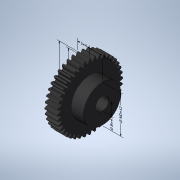
# Autodesk Inventor part: 21104000
Saved by Autodesk Inventor 2021 (Build 250183000, 183)
## iProperties
Created: 2025-12-15
Part Number: 21104000
Material: Generic
Catalog Web Link: www.3dfindit.com
Description: MAE-STZR-M0.5-MN-B4-ST-Spur Gears Made from Steel, with One-Sided Hub, Module 0.5, Tooth Width 4 mm
Vendor: MAEDLER
Document SubType Name: Modeling
Designer: psAdmin
Manufacturer: MAEDLER
Mass: 12 g
Surface Area: 13.391 cm^2
Volume: 1.60041 cm^3
Density: 1 g/cm^3
Appearance: PSOLRGB-176-176-176
Category: PARTsolutions
Company: MAEDLER
Title: 21104000
Author: Cadenas PARTsolutions
Comments: Spur Gears Made from Steel, with One-Sided Hub, Module 0.5, Tooth Width 4 mm
PSOL_IDENT_0: {$CADENAS_DATA/23d-libs/maedler/antriebselemente/stirnzahnraeder/stirnzahnraeder_stahl/modul_0_5_und
PSOL_IDENT_1: _0_7/stzr_m_0_5_zb4_st_mn.prj},173 {VTYP=3D},{NB=21104000},{LINA=21104000},{NN=MAE-STZR-M0.5-MN-B4-S
PSOL_IDENT_2: T},{DATE=31.10.2024 07:34:43},{GEOMDATE=31.10.2024 07:34:43},{VERSION=},{LINEID=240},{WBVAR=},{WBNUM
PSOL_IDENT_3: ERIC=}  {NB=21104000},{LINA=21104000},{KT=DUMMY},{ARTNR=21104000},{WEBSHOP=Produktdetails / Katalogs
PSOL_IDENT_4: eite / Montageanleitung},{MATK=Stahl},{MAT=Stahl 11SMn30+C (1.0715)},{M=0.5},{Z=40},{B=4},{DA=21.0},
PSOL_IDENT_5: {D=20.0},{NL=4},{ND=12},{BH7=4},{MD=10.3},{GEW=12.0},{CTN=84839089},{DIST=0.967},{GKD=18.79385},{FKD=
PSOL_IDENT_6: 18.83300},{T0=1.57080},{UF=62.83185},{TLG=1.57080},{A=3.42020},{A3=1.14007},{PI=0.39270},{R2=0.04},{
PSOL_IDENT_7: CNSDWTEMPLATE=_dw/ansicht_right_front.dw}
NB: 21104000
NN: MAE-STZR-M0.5-MN-B4-ST
NT: Spur Gears Made from Steel, with One-Sided Hub, Module 0.5, Tooth Width 4 mm
NBSYN: $ARTNR.
LINA: 21104000
CATALOG: MÄDLER
ARTNR: 21104000
WEBSHOP: Product details / Catalogue page / Assembly instructions
MATK: Steel
MAT: Steel 11SMn30+C (1.0715)
M: 0.5
Z: 40
B: 4
DA: 21
D: 20
NL: 4
ND: 12
BH7: 4
MD: 10.3
GEW: 12
CTN: 84839089
SUPPLIER: MAEDLER
ARTICLENO: 21104000
BOMINFO: 21104000
CREATOR: CADENAS GmbH
Autodesk Inventor part; units mm, degrees
ref_plane "YZ Plane" through (0, 0, 0) normal (1, 0, 0) x (0, 1, 0)
ref_plane "XZ Plane" through (0, 0, 0) normal (0, 1, 0) x (-1, 0, 0)
ref_plane "XY Plane" through (0, 0, 0) normal (0, 0, 1) x (1, 0, 0)
sketch "Sketch_2" plane through (0, 0, 0) normal (0, 0, 1) x (1, 0, 0)
  line L0 (6, 0) -> (-2, 0)
  line L1 (-2, 10.5) -> (-2, 2.1414)
  line L2 (-2, 2.1414) -> (-1.8586, 2)
  line L3 (-1.8586, 2) -> (5.8586, 2)
  line L4 (5.8586, 2) -> (6, 2.1414)
  line L5 (6, 2.1414) -> (6, 5.8586)
  line L6 (6, 5.8586) -> (5.8586, 6)
  line L7 (5.8586, 6) -> (2.1, 6)
  arc A0 (2, 6.1) -> (2.1, 6) centre (2.1, 6.1) ccw
  line L8 (2, 6.1) -> (2, 10.5)
  line L9 (2, 10.5) -> (-2, 10.5)
  constraints: 20 end point, 2 point on circle, 1 centre point
revolve "Revolution1" add sketch "Sketch_2" angle 360 about axis through (6, 0, 0) along (1, 0, 0)
sketch "Sketch_4" plane through (0, 0, 0) normal (1, 0, 0) x (0, 0, -1)
  circle A0 centre (0, 0) radius 21
  arc A1 (-10.4983, 0.1884) -> (-10.4983, -0.1884) centre (0, 0) ccw
  arc A2 (-10.4983, -0.1884) -> (-10.1352, -0.3434) centre (-8.8221, 3.2362) ccw
  arc A3 (-10.1352, -0.3434) -> (-9.9923, -0.3926) centre (-8.9496, 2.8648) ccw
  arc A4 (-9.9923, -0.3926) -> (-9.4352, -0.5161) centre (-9.0615, 2.4884) ccw
  arc A5 (-9.4002, -0.5534) -> (-9.4352, -0.5161) centre (-9.4402, -0.5558) ccw
  arc A6 (-9.4002, -0.5534) -> (-9.3711, -0.9239) centre (0, 0) ccw
  arc A7 (-9.3998, -0.9663) -> (-9.3711, -0.9239) centre (-9.4109, -0.9278) ccw
  arc A8 (-9.3998, -0.9663) -> (-9.9307, -1.1754) centre (-8.5606, -3.8753) ccw
  arc A9 (-9.9307, -1.1754) -> (-10.0641, -1.2464) centre (-8.3913, -4.2295) ccw
  arc A10 (-10.0641, -1.2464) -> (-10.3985, -1.4562) centre (-8.2072, -4.5764) ccw
  arc A11 (-10.3985, -1.4562) -> (-10.3396, -1.8283) centre (0, 0) ccw
  arc A12 (-10.3396, -1.8283) -> (-9.9567, -1.9246) centre (-9.2197, 1.8163) ccw
  arc A13 (-9.9567, -1.9246) -> (-9.8079, -1.9509) centre (-9.2876, 1.4295) ccw
  arc A14 (-9.8079, -1.9509) -> (-9.2383, -1.9857) centre (-9.3392, 1.0402) ccw
  arc A15 (-9.1979, -2.0171) -> (-9.2383, -1.9857) centre (-9.237, -2.0257) ccw
  arc A16 (-9.1979, -2.0171) -> (-9.1112, -2.3785) centre (0, 0) ccw
  arc A17 (-9.1329, -2.4248) -> (-9.1112, -2.3785) centre (-9.1499, -2.3886) ccw
  arc A18 (-9.1329, -2.4248) -> (-9.6246, -2.7144) centre (-7.849, -5.1667) ccw
  arc A19 (-9.6246, -2.7144) -> (-9.7452, -2.8054) centre (-7.6263, -5.4902) ccw
  arc A20 (-9.7452, -2.8054) -> (-10.0427, -3.065) centre (-7.3903, -5.804) ccw
  arc A21 (-10.0427, -3.065) -> (-9.9263, -3.4233) centre (0, 0) ccw
  arc A22 (-9.9263, -3.4233) -> (-9.533, -3.4585) centre (-9.3903, 0.3516) ccw
  arc A23 (-9.533, -3.4585) -> (-9.3819, -3.4612) centre (-9.3968, -0.041) ccw
  arc A24 (-9.3819, -3.4612) -> (-8.8139, -3.4065) centre (-9.3869, -0.4336) ccw
  arc A25 (-8.7691, -3.4312) -> (-8.8139, -3.4065) centre (-8.8064, -3.4457) ccw
  arc A26 (-8.7691, -3.4312) -> (-8.6269, -3.7745) centre (0, 0) ccw
  arc A27 (-8.6411, -3.8237) -> (-8.6269, -3.7745) centre (-8.6636, -3.7905) ccw
  arc A28 (-8.6411, -3.8237) -> (-9.0814, -4.1866) centre (-6.9441, -6.331) ccw
  arc A29 (-9.0814, -4.1866) -> (-9.1864, -4.2953) centre (-6.6736, -6.6156) ccw
  arc A30 (-9.1864, -4.2953) -> (-9.4396, -4.5983) centre (-6.3913, -6.8886) ccw
  arc A31 (-9.4396, -4.5983) -> (-9.2685, -4.934) centre (0, 0) ccw
  arc A32 (-9.2685, -4.934) -> (-8.8746, -4.9072) centre (-9.3297, -1.1217) ccw
  arc A33 (-8.8746, -4.9072) -> (-8.725, -4.8862) centre (-9.2747, -1.5105) ccw
  arc A34 (-8.725, -4.8862) -> (-8.1725, -4.7433) centre (-9.2035, -1.8967) ccw
  arc A35 (-8.1244, -4.7607) -> (-8.1725, -4.7433) centre (-8.1589, -4.7809) ccw
  arc A36 (-8.1244, -4.7607) -> (-7.9302, -5.0776) centre (0, 0) ccw
  arc A37 (-7.9366, -5.1284) -> (-7.9302, -5.0776) centre (-7.9639, -5.0992) ccw
  arc A38 (-7.9366, -5.1284) -> (-8.3147, -5.5557) centre (-5.8683, -7.3393) ccw
  arc A39 (-8.3147, -5.5557) -> (-8.4013, -5.6795) centre (-5.5565, -7.5781) ccw
  arc A40 (-8.4013, -5.6795) -> (-8.604, -6.0184) centre (-5.235, -7.8036) ccw
  arc A41 (-8.604, -6.0184) -> (-8.3826, -6.3231) centre (0, 0) ccw
  arc A42 (-8.3826, -6.3231) -> (-7.9977, -6.2351) centre (-9.0394, -2.5673) ccw
  arc A43 (-7.9977, -6.2351) -> (-7.8532, -6.1909) centre (-8.9243, -2.9428) ccw
  arc A44 (-7.8532, -6.1909) -> (-7.3299, -5.9634) centre (-8.7935, -3.3131) ccw
  arc A45 (-7.2796, -5.973) -> (-7.3299, -5.9634) centre (-7.3106, -5.9984) ccw
  arc A46 (-7.2796, -5.973) -> (-7.0383, -6.2556) centre (0, 0) ccw
  arc A47 (-7.0366, -6.3068) -> (-7.0383, -6.2556) centre (-7.0682, -6.2822) ccw
  arc A48 (-7.0366, -6.3068) -> (-7.3432, -6.788) centre (-4.6479, -8.167) ccw
  arc A49 (-7.3432, -6.788) -> (-7.4094, -6.9239) centre (-4.3026, -8.354) ccw
  arc A50 (-7.4094, -6.9239) -> (-7.5566, -7.2902) centre (-3.9498, -8.5265) ccw
  arc A51 (-7.5566, -7.2902) -> (-7.2902, -7.5566) centre (0, 0) ccw
  arc A52 (-7.2902, -7.5566) -> (-6.9239, -7.4094) centre (-8.5265, -3.9498) ccw
  arc A53 (-6.9239, -7.4094) -> (-6.788, -7.3432) centre (-8.354, -4.3026) ccw
  arc A54 (-6.788, -7.3432) -> (-6.3068, -7.0366) centre (-8.167, -4.6479) ccw
  arc A55 (-6.2556, -7.0383) -> (-6.3068, -7.0366) centre (-6.2822, -7.0682) ccw
  arc A56 (-6.2556, -7.0383) -> (-5.973, -7.2796) centre (0, 0) ccw
  arc A57 (-5.9634, -7.3299) -> (-5.973, -7.2796) centre (-5.9984, -7.3106) ccw
  arc A58 (-5.9634, -7.3299) -> (-6.1909, -7.8532) centre (-3.3131, -8.7935) ccw
  arc A59 (-6.1909, -7.8532) -> (-6.2351, -7.9977) centre (-2.9428, -8.9243) ccw
  arc A60 (-6.2351, -7.9977) -> (-6.3231, -8.3826) centre (-2.5673, -9.0394) ccw
  arc A61 (-6.3231, -8.3826) -> (-6.0184, -8.604) centre (0, 0) ccw
  arc A62 (-6.0184, -8.604) -> (-5.6795, -8.4013) centre (-7.8036, -5.235) ccw
  arc A63 (-5.6795, -8.4013) -> (-5.5557, -8.3147) centre (-7.5781, -5.5565) ccw
  arc A64 (-5.5557, -8.3147) -> (-5.1284, -7.9366) centre (-7.3393, -5.8683) ccw
  arc A65 (-5.0776, -7.9302) -> (-5.1284, -7.9366) centre (-5.0992, -7.9639) ccw
  arc A66 (-5.0776, -7.9302) -> (-4.7607, -8.1244) centre (0, 0) ccw
  arc A67 (-4.7433, -8.1725) -> (-4.7607, -8.1244) centre (-4.7809, -8.1589) ccw
  arc A68 (-4.7433, -8.1725) -> (-4.8862, -8.725) centre (-1.8967, -9.2035) ccw
  arc A69 (-4.8862, -8.725) -> (-4.9072, -8.8746) centre (-1.5105, -9.2747) ccw
  arc A70 (-4.9072, -8.8746) -> (-4.934, -9.2685) centre (-1.1217, -9.3297) ccw
  arc A71 (-4.934, -9.2685) -> (-4.5983, -9.4396) centre (0, 0) ccw
  arc A72 (-4.5983, -9.4396) -> (-4.2953, -9.1864) centre (-6.8886, -6.3913) ccw
  arc A73 (-4.2953, -9.1864) -> (-4.1866, -9.0814) centre (-6.6156, -6.6736) ccw
  arc A74 (-4.1866, -9.0814) -> (-3.8237, -8.6411) centre (-6.331, -6.9441) ccw
  arc A75 (-3.7745, -8.6269) -> (-3.8237, -8.6411) centre (-3.7905, -8.6636) ccw
  arc A76 (-3.7745, -8.6269) -> (-3.4312, -8.7691) centre (0, 0) ccw
  arc A77 (-3.4065, -8.8139) -> (-3.4312, -8.7691) centre (-3.4457, -8.8064) ccw
  arc A78 (-3.4065, -8.8139) -> (-3.4612, -9.3819) centre (-0.4336, -9.3869) ccw
  arc A79 (-3.4612, -9.3819) -> (-3.4585, -9.533) centre (-0.041, -9.3968) ccw
  arc A80 (-3.4585, -9.533) -> (-3.4233, -9.9263) centre (0.3516, -9.3903) ccw
  arc A81 (-3.4233, -9.9263) -> (-3.065, -10.0427) centre (0, 0) ccw
  arc A82 (-3.065, -10.0427) -> (-2.8054, -9.7452) centre (-5.804, -7.3903) ccw
  arc A83 (-2.8054, -9.7452) -> (-2.7144, -9.6246) centre (-5.4902, -7.6263) ccw
  arc A84 (-2.7144, -9.6246) -> (-2.4248, -9.1329) centre (-5.1667, -7.849) ccw
  arc A85 (-2.3785, -9.1112) -> (-2.4248, -9.1329) centre (-2.3886, -9.1499) ccw
  arc A86 (-2.3785, -9.1112) -> (-2.0171, -9.1979) centre (0, 0) ccw
  arc A87 (-1.9857, -9.2383) -> (-2.0171, -9.1979) centre (-2.0257, -9.237) ccw
  arc A88 (-1.9857, -9.2383) -> (-1.9509, -9.8079) centre (1.0402, -9.3392) ccw
  arc A89 (-1.9509, -9.8079) -> (-1.9246, -9.9567) centre (1.4295, -9.2876) ccw
  arc A90 (-1.9246, -9.9567) -> (-1.8283, -10.3396) centre (1.8163, -9.2197) ccw
  arc A91 (-1.8283, -10.3396) -> (-1.4562, -10.3985) centre (0, 0) ccw
  arc A92 (-1.4562, -10.3985) -> (-1.2464, -10.0641) centre (-4.5764, -8.2072) ccw
  arc A93 (-1.2464, -10.0641) -> (-1.1754, -9.9307) centre (-4.2295, -8.3913) ccw
  arc A94 (-1.1754, -9.9307) -> (-0.9663, -9.3998) centre (-3.8753, -8.5606) ccw
  arc A95 (-0.9239, -9.3711) -> (-0.9663, -9.3998) centre (-0.9278, -9.4109) ccw
  arc A96 (-0.9239, -9.3711) -> (-0.5534, -9.4002) centre (0, 0) ccw
  arc A97 (-0.5161, -9.4352) -> (-0.5534, -9.4002) centre (-0.5558, -9.4402) ccw
  arc A98 (-0.5161, -9.4352) -> (-0.3926, -9.9923) centre (2.4884, -9.0615) ccw
  arc A99 (-0.3926, -9.9923) -> (-0.3434, -10.1352) centre (2.8648, -8.9496) ccw
  arc A100 (-0.3434, -10.1352) -> (-0.1884, -10.4983) centre (3.2362, -8.8221) ccw
  arc A101 (-0.1884, -10.4983) -> (0.1884, -10.4983) centre (0, 0) ccw
  arc A102 (0.1884, -10.4983) -> (0.3434, -10.1352) centre (-3.2362, -8.8221) ccw
  arc A103 (0.3434, -10.1352) -> (0.3926, -9.9923) centre (-2.8648, -8.9496) ccw
  arc A104 (0.3926, -9.9923) -> (0.5161, -9.4352) centre (-2.4884, -9.0615) ccw
  arc A105 (0.5534, -9.4002) -> (0.5161, -9.4352) centre (0.5558, -9.4402) ccw
  arc A106 (0.5534, -9.4002) -> (0.9239, -9.3711) centre (0, 0) ccw
  arc A107 (0.9663, -9.3998) -> (0.9239, -9.3711) centre (0.9278, -9.4109) ccw
  arc A108 (0.9663, -9.3998) -> (1.1754, -9.9307) centre (3.8753, -8.5606) ccw
  arc A109 (1.1754, -9.9307) -> (1.2464, -10.0641) centre (4.2295, -8.3913) ccw
  arc A110 (1.2464, -10.0641) -> (1.4562, -10.3985) centre (4.5764, -8.2072) ccw
  arc A111 (1.4562, -10.3985) -> (1.8283, -10.3396) centre (0, 0) ccw
  arc A112 (1.8283, -10.3396) -> (1.9246, -9.9567) centre (-1.8163, -9.2197) ccw
  arc A113 (1.9246, -9.9567) -> (1.9509, -9.8079) centre (-1.4295, -9.2876) ccw
  arc A114 (1.9509, -9.8079) -> (1.9857, -9.2383) centre (-1.0402, -9.3392) ccw
  arc A115 (2.0171, -9.1979) -> (1.9857, -9.2383) centre (2.0257, -9.237) ccw
  arc A116 (2.0171, -9.1979) -> (2.3785, -9.1112) centre (0, 0) ccw
  arc A117 (2.4248, -9.1329) -> (2.3785, -9.1112) centre (2.3886, -9.1499) ccw
  arc A118 (2.4248, -9.1329) -> (2.7144, -9.6246) centre (5.1667, -7.849) ccw
  arc A119 (2.7144, -9.6246) -> (2.8054, -9.7452) centre (5.4902, -7.6263) ccw
  arc A120 (2.8054, -9.7452) -> (3.065, -10.0427) centre (5.804, -7.3903) ccw
  arc A121 (3.065, -10.0427) -> (3.4233, -9.9263) centre (0, 0) ccw
  arc A122 (3.4233, -9.9263) -> (3.4585, -9.533) centre (-0.3516, -9.3903) ccw
  arc A123 (3.4585, -9.533) -> (3.4612, -9.3819) centre (0.041, -9.3968) ccw
  arc A124 (3.4612, -9.3819) -> (3.4065, -8.8139) centre (0.4336, -9.3869) ccw
  arc A125 (3.4312, -8.7691) -> (3.4065, -8.8139) centre (3.4457, -8.8064) ccw
  arc A126 (3.4312, -8.7691) -> (3.7745, -8.6269) centre (0, 0) ccw
  arc A127 (3.8237, -8.6411) -> (3.7745, -8.6269) centre (3.7905, -8.6636) ccw
  arc A128 (3.8237, -8.6411) -> (4.1866, -9.0814) centre (6.331, -6.9441) ccw
  arc A129 (4.1866, -9.0814) -> (4.2953, -9.1864) centre (6.6156, -6.6736) ccw
  arc A130 (4.2953, -9.1864) -> (4.5983, -9.4396) centre (6.8886, -6.3913) ccw
  arc A131 (4.5983, -9.4396) -> (4.934, -9.2685) centre (0, 0) ccw
  arc A132 (4.934, -9.2685) -> (4.9072, -8.8746) centre (1.1217, -9.3297) ccw
  arc A133 (4.9072, -8.8746) -> (4.8862, -8.725) centre (1.5105, -9.2747) ccw
  arc A134 (4.8862, -8.725) -> (4.7433, -8.1725) centre (1.8967, -9.2035) ccw
  arc A135 (4.7607, -8.1244) -> (4.7433, -8.1725) centre (4.7809, -8.1589) ccw
  arc A136 (4.7607, -8.1244) -> (5.0776, -7.9302) centre (0, 0) ccw
  arc A137 (5.1284, -7.9366) -> (5.0776, -7.9302) centre (5.0992, -7.9639) ccw
  arc A138 (5.1284, -7.9366) -> (5.5557, -8.3147) centre (7.3393, -5.8683) ccw
  arc A139 (5.5557, -8.3147) -> (5.6795, -8.4013) centre (7.5781, -5.5565) ccw
  arc A140 (5.6795, -8.4013) -> (6.0184, -8.604) centre (7.8036, -5.235) ccw
  arc A141 (6.0184, -8.604) -> (6.3231, -8.3826) centre (0, 0) ccw
  arc A142 (6.3231, -8.3826) -> (6.2351, -7.9977) centre (2.5673, -9.0394) ccw
  arc A143 (6.2351, -7.9977) -> (6.1909, -7.8532) centre (2.9428, -8.9243) ccw
  arc A144 (6.1909, -7.8532) -> (5.9634, -7.3299) centre (3.3131, -8.7935) ccw
  arc A145 (5.973, -7.2796) -> (5.9634, -7.3299) centre (5.9984, -7.3106) ccw
  arc A146 (5.973, -7.2796) -> (6.2556, -7.0383) centre (0, 0) ccw
  arc A147 (6.3068, -7.0366) -> (6.2556, -7.0383) centre (6.2822, -7.0682) ccw
  arc A148 (6.3068, -7.0366) -> (6.788, -7.3432) centre (8.167, -4.6479) ccw
  arc A149 (6.788, -7.3432) -> (6.9239, -7.4094) centre (8.354, -4.3026) ccw
  arc A150 (6.9239, -7.4094) -> (7.2902, -7.5566) centre (8.5265, -3.9498) ccw
  arc A151 (7.2902, -7.5566) -> (7.5566, -7.2902) centre (0, 0) ccw
  arc A152 (7.5566, -7.2902) -> (7.4094, -6.9239) centre (3.9498, -8.5265) ccw
  arc A153 (7.4094, -6.9239) -> (7.3432, -6.788) centre (4.3026, -8.354) ccw
  arc A154 (7.3432, -6.788) -> (7.0366, -6.3068) centre (4.6479, -8.167) ccw
  arc A155 (7.0383, -6.2556) -> (7.0366, -6.3068) centre (7.0682, -6.2822) ccw
  arc A156 (7.0383, -6.2556) -> (7.2796, -5.973) centre (0, 0) ccw
  arc A157 (7.3299, -5.9634) -> (7.2796, -5.973) centre (7.3106, -5.9984) ccw
  arc A158 (7.3299, -5.9634) -> (7.8532, -6.1909) centre (8.7935, -3.3131) ccw
  arc A159 (7.8532, -6.1909) -> (7.9977, -6.2351) centre (8.9243, -2.9428) ccw
  arc A160 (7.9977, -6.2351) -> (8.3826, -6.3231) centre (9.0394, -2.5673) ccw
  arc A161 (8.3826, -6.3231) -> (8.604, -6.0184) centre (0, 0) ccw
  arc A162 (8.604, -6.0184) -> (8.4013, -5.6795) centre (5.235, -7.8036) ccw
  arc A163 (8.4013, -5.6795) -> (8.3147, -5.5557) centre (5.5565, -7.5781) ccw
  arc A164 (8.3147, -5.5557) -> (7.9366, -5.1284) centre (5.8683, -7.3393) ccw
  arc A165 (7.9302, -5.0776) -> (7.9366, -5.1284) centre (7.9639, -5.0992) ccw
  arc A166 (7.9302, -5.0776) -> (8.1244, -4.7607) centre (0, 0) ccw
  arc A167 (8.1725, -4.7433) -> (8.1244, -4.7607) centre (8.1589, -4.7809) ccw
  arc A168 (8.1725, -4.7433) -> (8.725, -4.8862) centre (9.2035, -1.8967) ccw
  arc A169 (8.725, -4.8862) -> (8.8746, -4.9072) centre (9.2747, -1.5105) ccw
  arc A170 (8.8746, -4.9072) -> (9.2685, -4.934) centre (9.3297, -1.1217) ccw
  arc A171 (9.2685, -4.934) -> (9.4396, -4.5983) centre (0, 0) ccw
  arc A172 (9.4396, -4.5983) -> (9.1864, -4.2953) centre (6.3913, -6.8886) ccw
  arc A173 (9.1864, -4.2953) -> (9.0814, -4.1866) centre (6.6736, -6.6156) ccw
  arc A174 (9.0814, -4.1866) -> (8.6411, -3.8237) centre (6.9441, -6.331) ccw
  arc A175 (8.6269, -3.7745) -> (8.6411, -3.8237) centre (8.6636, -3.7905) ccw
  arc A176 (8.6269, -3.7745) -> (8.7691, -3.4312) centre (0, 0) ccw
  arc A177 (8.8139, -3.4065) -> (8.7691, -3.4312) centre (8.8064, -3.4457) ccw
  arc A178 (8.8139, -3.4065) -> (9.3819, -3.4612) centre (9.3869, -0.4336) ccw
  arc A179 (9.3819, -3.4612) -> (9.533, -3.4585) centre (9.3968, -0.041) ccw
  arc A180 (9.533, -3.4585) -> (9.9263, -3.4233) centre (9.3903, 0.3516) ccw
  arc A181 (9.9263, -3.4233) -> (10.0427, -3.065) centre (0, 0) ccw
  arc A182 (10.0427, -3.065) -> (9.7452, -2.8054) centre (7.3903, -5.804) ccw
  arc A183 (9.7452, -2.8054) -> (9.6246, -2.7144) centre (7.6263, -5.4902) ccw
  arc A184 (9.6246, -2.7144) -> (9.1329, -2.4248) centre (7.849, -5.1667) ccw
  arc A185 (9.1112, -2.3785) -> (9.1329, -2.4248) centre (9.1499, -2.3886) ccw
  arc A186 (9.1112, -2.3785) -> (9.1979, -2.0171) centre (0, 0) ccw
  arc A187 (9.2383, -1.9857) -> (9.1979, -2.0171) centre (9.237, -2.0257) ccw
  arc A188 (9.2383, -1.9857) -> (9.8079, -1.9509) centre (9.3392, 1.0402) ccw
  arc A189 (9.8079, -1.9509) -> (9.9567, -1.9246) centre (9.2876, 1.4295) ccw
  arc A190 (9.9567, -1.9246) -> (10.3396, -1.8283) centre (9.2197, 1.8163) ccw
  arc A191 (10.3396, -1.8283) -> (10.3985, -1.4562) centre (0, 0) ccw
  arc A192 (10.3985, -1.4562) -> (10.0641, -1.2464) centre (8.2072, -4.5764) ccw
  arc A193 (10.0641, -1.2464) -> (9.9307, -1.1754) centre (8.3913, -4.2295) ccw
  arc A194 (9.9307, -1.1754) -> (9.3998, -0.9663) centre (8.5606, -3.8753) ccw
  arc A195 (9.3711, -0.9239) -> (9.3998, -0.9663) centre (9.4109, -0.9278) ccw
  arc A196 (9.3711, -0.9239) -> (9.4002, -0.5534) centre (0, 0) ccw
  arc A197 (9.4352, -0.5161) -> (9.4002, -0.5534) centre (9.4402, -0.5558) ccw
  arc A198 (9.4352, -0.5161) -> (9.9923, -0.3926) centre (9.0615, 2.4884) ccw
  arc A199 (9.9923, -0.3926) -> (10.1352, -0.3434) centre (8.9496, 2.8648) ccw
  arc A200 (10.1352, -0.3434) -> (10.4983, -0.1884) centre (8.8221, 3.2362) ccw
  arc A201 (10.4983, -0.1884) -> (10.4983, 0.1884) centre (0, 0) ccw
  arc A202 (10.4983, 0.1884) -> (10.1352, 0.3434) centre (8.8221, -3.2362) ccw
  arc A203 (10.1352, 0.3434) -> (9.9923, 0.3926) centre (8.9496, -2.8648) ccw
  arc A204 (9.9923, 0.3926) -> (9.4352, 0.5161) centre (9.0615, -2.4884) ccw
  arc A205 (9.4002, 0.5534) -> (9.4352, 0.5161) centre (9.4402, 0.5558) ccw
  arc A206 (9.4002, 0.5534) -> (9.3711, 0.9239) centre (0, 0) ccw
  arc A207 (9.3998, 0.9663) -> (9.3711, 0.9239) centre (9.4109, 0.9278) ccw
  arc A208 (9.3998, 0.9663) -> (9.9307, 1.1754) centre (8.5606, 3.8753) ccw
  arc A209 (9.9307, 1.1754) -> (10.0641, 1.2464) centre (8.3913, 4.2295) ccw
  arc A210 (10.0641, 1.2464) -> (10.3985, 1.4562) centre (8.2072, 4.5764) ccw
  arc A211 (10.3985, 1.4562) -> (10.3396, 1.8283) centre (0, 0) ccw
  arc A212 (10.3396, 1.8283) -> (9.9567, 1.9246) centre (9.2197, -1.8163) ccw
  arc A213 (9.9567, 1.9246) -> (9.8079, 1.9509) centre (9.2876, -1.4295) ccw
  arc A214 (9.8079, 1.9509) -> (9.2383, 1.9857) centre (9.3392, -1.0402) ccw
  arc A215 (9.1979, 2.0171) -> (9.2383, 1.9857) centre (9.237, 2.0257) ccw
  arc A216 (9.1979, 2.0171) -> (9.1112, 2.3785) centre (0, 0) ccw
  arc A217 (9.1329, 2.4248) -> (9.1112, 2.3785) centre (9.1499, 2.3886) ccw
  arc A218 (9.1329, 2.4248) -> (9.6246, 2.7144) centre (7.849, 5.1667) ccw
  arc A219 (9.6246, 2.7144) -> (9.7452, 2.8054) centre (7.6263, 5.4902) ccw
  arc A220 (9.7452, 2.8054) -> (10.0427, 3.065) centre (7.3903, 5.804) ccw
  arc A221 (10.0427, 3.065) -> (9.9263, 3.4233) centre (0, 0) ccw
  arc A222 (9.9263, 3.4233) -> (9.533, 3.4585) centre (9.3903, -0.3516) ccw
  arc A223 (9.533, 3.4585) -> (9.3819, 3.4612) centre (9.3968, 0.041) ccw
  arc A224 (9.3819, 3.4612) -> (8.8139, 3.4065) centre (9.3869, 0.4336) ccw
  arc A225 (8.7691, 3.4312) -> (8.8139, 3.4065) centre (8.8064, 3.4457) ccw
  arc A226 (8.7691, 3.4312) -> (8.6269, 3.7745) centre (0, 0) ccw
  arc A227 (8.6411, 3.8237) -> (8.6269, 3.7745) centre (8.6636, 3.7905) ccw
  arc A228 (8.6411, 3.8237) -> (9.0814, 4.1866) centre (6.9441, 6.331) ccw
  arc A229 (9.0814, 4.1866) -> (9.1864, 4.2953) centre (6.6736, 6.6156) ccw
  arc A230 (9.1864, 4.2953) -> (9.4396, 4.5983) centre (6.3913, 6.8886) ccw
  arc A231 (9.4396, 4.5983) -> (9.2685, 4.934) centre (0, 0) ccw
  arc A232 (9.2685, 4.934) -> (8.8746, 4.9072) centre (9.3297, 1.1217) ccw
  arc A233 (8.8746, 4.9072) -> (8.725, 4.8862) centre (9.2747, 1.5105) ccw
  arc A234 (8.725, 4.8862) -> (8.1725, 4.7433) centre (9.2035, 1.8967) ccw
  arc A235 (8.1244, 4.7607) -> (8.1725, 4.7433) centre (8.1589, 4.7809) ccw
  arc A236 (8.1244, 4.7607) -> (7.9302, 5.0776) centre (0, 0) ccw
  arc A237 (7.9366, 5.1284) -> (7.9302, 5.0776) centre (7.9639, 5.0992) ccw
  arc A238 (7.9366, 5.1284) -> (8.3147, 5.5557) centre (5.8683, 7.3393) ccw
  arc A239 (8.3147, 5.5557) -> (8.4013, 5.6795) centre (5.5565, 7.5781) ccw
  arc A240 (8.4013, 5.6795) -> (8.604, 6.0184) centre (5.235, 7.8036) ccw
  arc A241 (8.604, 6.0184) -> (8.3826, 6.3231) centre (0, 0) ccw
  arc A242 (8.3826, 6.3231) -> (7.9977, 6.2351) centre (9.0394, 2.5673) ccw
  arc A243 (7.9977, 6.2351) -> (7.8532, 6.1909) centre (8.9243, 2.9428) ccw
  arc A244 (7.8532, 6.1909) -> (7.3299, 5.9634) centre (8.7935, 3.3131) ccw
  arc A245 (7.2796, 5.973) -> (7.3299, 5.9634) centre (7.3106, 5.9984) ccw
  arc A246 (7.2796, 5.973) -> (7.0383, 6.2556) centre (0, 0) ccw
  arc A247 (7.0366, 6.3068) -> (7.0383, 6.2556) centre (7.0682, 6.2822) ccw
  arc A248 (7.0366, 6.3068) -> (7.3432, 6.788) centre (4.6479, 8.167) ccw
  arc A249 (7.3432, 6.788) -> (7.4094, 6.9239) centre (4.3026, 8.354) ccw
  arc A250 (7.4094, 6.9239) -> (7.5566, 7.2902) centre (3.9498, 8.5265) ccw
  arc A251 (7.5566, 7.2902) -> (7.2902, 7.5566) centre (0, 0) ccw
  arc A252 (7.2902, 7.5566) -> (6.9239, 7.4094) centre (8.5265, 3.9498) ccw
  arc A253 (6.9239, 7.4094) -> (6.788, 7.3432) centre (8.354, 4.3026) ccw
  arc A254 (6.788, 7.3432) -> (6.3068, 7.0366) centre (8.167, 4.6479) ccw
  arc A255 (6.2556, 7.0383) -> (6.3068, 7.0366) centre (6.2822, 7.0682) ccw
  arc A256 (6.2556, 7.0383) -> (5.973, 7.2796) centre (0, 0) ccw
  arc A257 (5.9634, 7.3299) -> (5.973, 7.2796) centre (5.9984, 7.3106) ccw
  arc A258 (5.9634, 7.3299) -> (6.1909, 7.8532) centre (3.3131, 8.7935) ccw
  arc A259 (6.1909, 7.8532) -> (6.2351, 7.9977) centre (2.9428, 8.9243) ccw
  arc A260 (6.2351, 7.9977) -> (6.3231, 8.3826) centre (2.5673, 9.0394) ccw
  arc A261 (6.3231, 8.3826) -> (6.0184, 8.604) centre (0, 0) ccw
  arc A262 (6.0184, 8.604) -> (5.6795, 8.4013) centre (7.8036, 5.235) ccw
  arc A263 (5.6795, 8.4013) -> (5.5557, 8.3147) centre (7.5781, 5.5565) ccw
  arc A264 (5.5557, 8.3147) -> (5.1284, 7.9366) centre (7.3393, 5.8683) ccw
  arc A265 (5.0776, 7.9302) -> (5.1284, 7.9366) centre (5.0992, 7.9639) ccw
  arc A266 (5.0776, 7.9302) -> (4.7607, 8.1244) centre (0, 0) ccw
  arc A267 (4.7433, 8.1725) -> (4.7607, 8.1244) centre (4.7809, 8.1589) ccw
  arc A268 (4.7433, 8.1725) -> (4.8862, 8.725) centre (1.8967, 9.2035) ccw
  arc A269 (4.8862, 8.725) -> (4.9072, 8.8746) centre (1.5105, 9.2747) ccw
  arc A270 (4.9072, 8.8746) -> (4.934, 9.2685) centre (1.1217, 9.3297) ccw
  arc A271 (4.934, 9.2685) -> (4.5983, 9.4396) centre (0, 0) ccw
  arc A272 (4.5983, 9.4396) -> (4.2953, 9.1864) centre (6.8886, 6.3913) ccw
  arc A273 (4.2953, 9.1864) -> (4.1866, 9.0814) centre (6.6156, 6.6736) ccw
  arc A274 (4.1866, 9.0814) -> (3.8237, 8.6411) centre (6.331, 6.9441) ccw
  arc A275 (3.7745, 8.6269) -> (3.8237, 8.6411) centre (3.7905, 8.6636) ccw
  arc A276 (3.7745, 8.6269) -> (3.4312, 8.7691) centre (0, 0) ccw
  arc A277 (3.4065, 8.8139) -> (3.4312, 8.7691) centre (3.4457, 8.8064) ccw
  arc A278 (3.4065, 8.8139) -> (3.4612, 9.3819) centre (0.4336, 9.3869) ccw
  arc A279 (3.4612, 9.3819) -> (3.4585, 9.533) centre (0.041, 9.3968) ccw
  arc A280 (3.4585, 9.533) -> (3.4233, 9.9263) centre (-0.3516, 9.3903) ccw
  arc A281 (3.4233, 9.9263) -> (3.065, 10.0427) centre (0, 0) ccw
  arc A282 (3.065, 10.0427) -> (2.8054, 9.7452) centre (5.804, 7.3903) ccw
  arc A283 (2.8054, 9.7452) -> (2.7144, 9.6246) centre (5.4902, 7.6263) ccw
  arc A284 (2.7144, 9.6246) -> (2.4248, 9.1329) centre (5.1667, 7.849) ccw
  arc A285 (2.3785, 9.1112) -> (2.4248, 9.1329) centre (2.3886, 9.1499) ccw
  arc A286 (2.3785, 9.1112) -> (2.0171, 9.1979) centre (0, 0) ccw
  arc A287 (1.9857, 9.2383) -> (2.0171, 9.1979) centre (2.0257, 9.237) ccw
  arc A288 (1.9857, 9.2383) -> (1.9509, 9.8079) centre (-1.0402, 9.3392) ccw
  arc A289 (1.9509, 9.8079) -> (1.9246, 9.9567) centre (-1.4295, 9.2876) ccw
  arc A290 (1.9246, 9.9567) -> (1.8283, 10.3396) centre (-1.8163, 9.2197) ccw
  arc A291 (1.8283, 10.3396) -> (1.4562, 10.3985) centre (0, 0) ccw
  arc A292 (1.4562, 10.3985) -> (1.2464, 10.0641) centre (4.5764, 8.2072) ccw
  arc A293 (1.2464, 10.0641) -> (1.1754, 9.9307) centre (4.2295, 8.3913) ccw
  arc A294 (1.1754, 9.9307) -> (0.9663, 9.3998) centre (3.8753, 8.5606) ccw
  arc A295 (0.9239, 9.3711) -> (0.9663, 9.3998) centre (0.9278, 9.4109) ccw
  arc A296 (0.9239, 9.3711) -> (0.5534, 9.4002) centre (0, 0) ccw
  arc A297 (0.5161, 9.4352) -> (0.5534, 9.4002) centre (0.5558, 9.4402) ccw
  arc A298 (0.5161, 9.4352) -> (0.3926, 9.9923) centre (-2.4884, 9.0615) ccw
  arc A299 (0.3926, 9.9923) -> (0.3434, 10.1352) centre (-2.8648, 8.9496) ccw
  arc A300 (0.3434, 10.1352) -> (0.1884, 10.4983) centre (-3.2362, 8.8221) ccw
  arc A301 (0.1884, 10.4983) -> (-0.1884, 10.4983) centre (0, 0) ccw
  arc A302 (-0.1884, 10.4983) -> (-0.3434, 10.1352) centre (3.2362, 8.8221) ccw
  arc A303 (-0.3434, 10.1352) -> (-0.3926, 9.9923) centre (2.8648, 8.9496) ccw
  arc A304 (-0.3926, 9.9923) -> (-0.5161, 9.4352) centre (2.4884, 9.0615) ccw
  arc A305 (-0.5534, 9.4002) -> (-0.5161, 9.4352) centre (-0.5558, 9.4402) ccw
  arc A306 (-0.5534, 9.4002) -> (-0.9239, 9.3711) centre (0, 0) ccw
  arc A307 (-0.9663, 9.3998) -> (-0.9239, 9.3711) centre (-0.9278, 9.4109) ccw
  arc A308 (-0.9663, 9.3998) -> (-1.1754, 9.9307) centre (-3.8753, 8.5606) ccw
  arc A309 (-1.1754, 9.9307) -> (-1.2464, 10.0641) centre (-4.2295, 8.3913) ccw
  arc A310 (-1.2464, 10.0641) -> (-1.4562, 10.3985) centre (-4.5764, 8.2072) ccw
  arc A311 (-1.4562, 10.3985) -> (-1.8283, 10.3396) centre (0, 0) ccw
  arc A312 (-1.8283, 10.3396) -> (-1.9246, 9.9567) centre (1.8163, 9.2197) ccw
  arc A313 (-1.9246, 9.9567) -> (-1.9509, 9.8079) centre (1.4295, 9.2876) ccw
  arc A314 (-1.9509, 9.8079) -> (-1.9857, 9.2383) centre (1.0402, 9.3392) ccw
  arc A315 (-2.0171, 9.1979) -> (-1.9857, 9.2383) centre (-2.0257, 9.237) ccw
  arc A316 (-2.0171, 9.1979) -> (-2.3785, 9.1112) centre (0, 0) ccw
  arc A317 (-2.4248, 9.1329) -> (-2.3785, 9.1112) centre (-2.3886, 9.1499) ccw
  arc A318 (-2.4248, 9.1329) -> (-2.7144, 9.6246) centre (-5.1667, 7.849) ccw
  arc A319 (-2.7144, 9.6246) -> (-2.8054, 9.7452) centre (-5.4902, 7.6263) ccw
  arc A320 (-2.8054, 9.7452) -> (-3.065, 10.0427) centre (-5.804, 7.3903) ccw
  arc A321 (-3.065, 10.0427) -> (-3.4233, 9.9263) centre (0, 0) ccw
  arc A322 (-3.4233, 9.9263) -> (-3.4585, 9.533) centre (0.3516, 9.3903) ccw
  arc A323 (-3.4585, 9.533) -> (-3.4612, 9.3819) centre (-0.041, 9.3968) ccw
  arc A324 (-3.4612, 9.3819) -> (-3.4065, 8.8139) centre (-0.4336, 9.3869) ccw
  arc A325 (-3.4312, 8.7691) -> (-3.4065, 8.8139) centre (-3.4457, 8.8064) ccw
  arc A326 (-3.4312, 8.7691) -> (-3.7745, 8.6269) centre (0, 0) ccw
  arc A327 (-3.8237, 8.6411) -> (-3.7745, 8.6269) centre (-3.7905, 8.6636) ccw
  arc A328 (-3.8237, 8.6411) -> (-4.1866, 9.0814) centre (-6.331, 6.9441) ccw
  arc A329 (-4.1866, 9.0814) -> (-4.2953, 9.1864) centre (-6.6156, 6.6736) ccw
  arc A330 (-4.2953, 9.1864) -> (-4.5983, 9.4396) centre (-6.8886, 6.3913) ccw
  arc A331 (-4.5983, 9.4396) -> (-4.934, 9.2685) centre (0, 0) ccw
  arc A332 (-4.934, 9.2685) -> (-4.9072, 8.8746) centre (-1.1217, 9.3297) ccw
  arc A333 (-4.9072, 8.8746) -> (-4.8862, 8.725) centre (-1.5105, 9.2747) ccw
  arc A334 (-4.8862, 8.725) -> (-4.7433, 8.1725) centre (-1.8967, 9.2035) ccw
  arc A335 (-4.7607, 8.1244) -> (-4.7433, 8.1725) centre (-4.7809, 8.1589) ccw
  arc A336 (-4.7607, 8.1244) -> (-5.0776, 7.9302) centre (0, 0) ccw
  arc A337 (-5.1284, 7.9366) -> (-5.0776, 7.9302) centre (-5.0992, 7.9639) ccw
  arc A338 (-5.1284, 7.9366) -> (-5.5557, 8.3147) centre (-7.3393, 5.8683) ccw
  arc A339 (-5.5557, 8.3147) -> (-5.6795, 8.4013) centre (-7.5781, 5.5565) ccw
  arc A340 (-5.6795, 8.4013) -> (-6.0184, 8.604) centre (-7.8036, 5.235) ccw
  arc A341 (-6.0184, 8.604) -> (-6.3231, 8.3826) centre (0, 0) ccw
  arc A342 (-6.3231, 8.3826) -> (-6.2351, 7.9977) centre (-2.5673, 9.0394) ccw
  arc A343 (-6.2351, 7.9977) -> (-6.1909, 7.8532) centre (-2.9428, 8.9243) ccw
  arc A344 (-6.1909, 7.8532) -> (-5.9634, 7.3299) centre (-3.3131, 8.7935) ccw
  arc A345 (-5.973, 7.2796) -> (-5.9634, 7.3299) centre (-5.9984, 7.3106) ccw
  arc A346 (-5.973, 7.2796) -> (-6.2556, 7.0383) centre (0, 0) ccw
  arc A347 (-6.3068, 7.0366) -> (-6.2556, 7.0383) centre (-6.2822, 7.0682) ccw
  arc A348 (-6.3068, 7.0366) -> (-6.788, 7.3432) centre (-8.167, 4.6479) ccw
  arc A349 (-6.788, 7.3432) -> (-6.9239, 7.4094) centre (-8.354, 4.3026) ccw
  arc A350 (-6.9239, 7.4094) -> (-7.2902, 7.5566) centre (-8.5265, 3.9498) ccw
  arc A351 (-7.2902, 7.5566) -> (-7.5566, 7.2902) centre (0, 0) ccw
  arc A352 (-7.5566, 7.2902) -> (-7.4094, 6.9239) centre (-3.9498, 8.5265) ccw
  arc A353 (-7.4094, 6.9239) -> (-7.3432, 6.788) centre (-4.3026, 8.354) ccw
  arc A354 (-7.3432, 6.788) -> (-7.0366, 6.3068) centre (-4.6479, 8.167) ccw
  arc A355 (-7.0383, 6.2556) -> (-7.0366, 6.3068) centre (-7.0682, 6.2822) ccw
  arc A356 (-7.0383, 6.2556) -> (-7.2796, 5.973) centre (0, 0) ccw
  arc A357 (-7.3299, 5.9634) -> (-7.2796, 5.973) centre (-7.3106, 5.9984) ccw
  arc A358 (-7.3299, 5.9634) -> (-7.8532, 6.1909) centre (-8.7935, 3.3131) ccw
  arc A359 (-7.8532, 6.1909) -> (-7.9977, 6.2351) centre (-8.9243, 2.9428) ccw
  arc A360 (-7.9977, 6.2351) -> (-8.3826, 6.3231) centre (-9.0394, 2.5673) ccw
  arc A361 (-8.3826, 6.3231) -> (-8.604, 6.0184) centre (0, 0) ccw
  arc A362 (-8.604, 6.0184) -> (-8.4013, 5.6795) centre (-5.235, 7.8036) ccw
  arc A363 (-8.4013, 5.6795) -> (-8.3147, 5.5557) centre (-5.5565, 7.5781) ccw
  arc A364 (-8.3147, 5.5557) -> (-7.9366, 5.1284) centre (-5.8683, 7.3393) ccw
  arc A365 (-7.9302, 5.0776) -> (-7.9366, 5.1284) centre (-7.9639, 5.0992) ccw
  arc A366 (-7.9302, 5.0776) -> (-8.1244, 4.7607) centre (0, 0) ccw
  arc A367 (-8.1725, 4.7433) -> (-8.1244, 4.7607) centre (-8.1589, 4.7809) ccw
  arc A368 (-8.1725, 4.7433) -> (-8.725, 4.8862) centre (-9.2035, 1.8967) ccw
  arc A369 (-8.725, 4.8862) -> (-8.8746, 4.9072) centre (-9.2747, 1.5105) ccw
  arc A370 (-8.8746, 4.9072) -> (-9.2685, 4.934) centre (-9.3297, 1.1217) ccw
  arc A371 (-9.2685, 4.934) -> (-9.4396, 4.5983) centre (0, 0) ccw
  arc A372 (-9.4396, 4.5983) -> (-9.1864, 4.2953) centre (-6.3913, 6.8886) ccw
  arc A373 (-9.1864, 4.2953) -> (-9.0814, 4.1866) centre (-6.6736, 6.6156) ccw
  arc A374 (-9.0814, 4.1866) -> (-8.6411, 3.8237) centre (-6.9441, 6.331) ccw
  arc A375 (-8.6269, 3.7745) -> (-8.6411, 3.8237) centre (-8.6636, 3.7905) ccw
  arc A376 (-8.6269, 3.7745) -> (-8.7691, 3.4312) centre (0, 0) ccw
  arc A377 (-8.8139, 3.4065) -> (-8.7691, 3.4312) centre (-8.8064, 3.4457) ccw
  arc A378 (-8.8139, 3.4065) -> (-9.3819, 3.4612) centre (-9.3869, 0.4336) ccw
  arc A379 (-9.3819, 3.4612) -> (-9.533, 3.4585) centre (-9.3968, 0.041) ccw
  arc A380 (-9.533, 3.4585) -> (-9.9263, 3.4233) centre (-9.3903, -0.3516) ccw
  arc A381 (-9.9263, 3.4233) -> (-10.0427, 3.065) centre (0, 0) ccw
  arc A382 (-10.0427, 3.065) -> (-9.7452, 2.8054) centre (-7.3903, 5.804) ccw
  arc A383 (-9.7452, 2.8054) -> (-9.6246, 2.7144) centre (-7.6263, 5.4902) ccw
  arc A384 (-9.6246, 2.7144) -> (-9.1329, 2.4248) centre (-7.849, 5.1667) ccw
  arc A385 (-9.1112, 2.3785) -> (-9.1329, 2.4248) centre (-9.1499, 2.3886) ccw
  arc A386 (-9.1112, 2.3785) -> (-9.1979, 2.0171) centre (0, 0) ccw
  arc A387 (-9.2383, 1.9857) -> (-9.1979, 2.0171) centre (-9.237, 2.0257) ccw
  arc A388 (-9.2383, 1.9857) -> (-9.8079, 1.9509) centre (-9.3392, -1.0402) ccw
  arc A389 (-9.8079, 1.9509) -> (-9.9567, 1.9246) centre (-9.2876, -1.4295) ccw
  arc A390 (-9.9567, 1.9246) -> (-10.3396, 1.8283) centre (-9.2197, -1.8163) ccw
  arc A391 (-10.3396, 1.8283) -> (-10.3985, 1.4562) centre (0, 0) ccw
  arc A392 (-10.3985, 1.4562) -> (-10.0641, 1.2464) centre (-8.2072, 4.5764) ccw
  arc A393 (-10.0641, 1.2464) -> (-9.9307, 1.1754) centre (-8.3913, 4.2295) ccw
  arc A394 (-9.9307, 1.1754) -> (-9.3998, 0.9663) centre (-8.5606, 3.8753) ccw
  arc A395 (-9.3711, 0.9239) -> (-9.3998, 0.9663) centre (-9.4109, 0.9278) ccw
  arc A396 (-9.3711, 0.9239) -> (-9.4002, 0.5534) centre (0, 0) ccw
  arc A397 (-9.4352, 0.5161) -> (-9.4002, 0.5534) centre (-9.4402, 0.5558) ccw
  arc A398 (-9.4352, 0.5161) -> (-9.9923, 0.3926) centre (-9.0615, -2.4884) ccw
  arc A399 (-9.9923, 0.3926) -> (-10.1352, 0.3434) centre (-8.9496, -2.8648) ccw
  arc A400 (-10.1352, 0.3434) -> (-10.4983, 0.1884) centre (-8.8221, -3.2362) ccw
  constraints: 800 point on circle, 401 centre point
extrude "Extrusion1" cut sketch "Sketch_4" along normal mid plane 4
body "Solid1"
